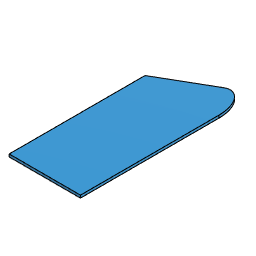
Nupud-T1 v1 (Autodesk Fusion 360 design; units mm, degrees)
Autodesk Fusion 360 part; units mm, degrees
sketch "Sketch1" plane through (0, 0, 0) normal (0, 0, 1) x (1, 0, 0)
  line L0 (-33, -71.5) -> (-33, -39.0517)
  spline S0 degree 3 poles (-33, -39.0517) (-33, -37.2602) (-33.4854, -35.4836) (-34.2537, -34.2725) (-34.9261, -33.2125) (-35.7722, -32.611) (-36.5563, -32.4575) (-37.1254, -32.346) (-37.6904, -32.44) (-38.2678, -32.7734) knots -1.570796 -1.570796 -1.570796 -1.570796 -0.801145 -0.801145 -0.801145 -0.12753 -0.12753 -0.12753 0.361367 0.361367 0.361367 0.361367
  line L1 (-38.2678, -32.7734) -> (-50, -39.547)
  line L2 (-50, -39.547) -> (-50, -71.5)
  line L3 (-50, -71.5) -> (-33, -71.5)
  line L4 (-33.2, -71.3) -> (-33.2, -39.0517)
  spline S1 degree 3 poles (-33.2, -39.0517) (-33.2, -37.2964) (-33.6813, -35.5482) (-34.4225, -34.3796) (-35.0726, -33.3548) (-35.8807, -32.7936) (-36.5947, -32.6537) (-37.1185, -32.5512) (-37.6252, -32.6333) (-38.1678, -32.9466) knots -1.570796 -1.570796 -1.570796 -1.570796 -0.801145 -0.801145 -0.801145 -0.12753 -0.12753 -0.12753 0.361367 0.361367 0.361367 0.361367
  line L5 (-38.1678, -32.9466) -> (-49.8, -39.6625)
  line L6 (-49.8, -39.6625) -> (-49.8, -71.3)
  line L7 (-49.8, -71.3) -> (-33.2, -71.3)
  dimension "d1" = 17
  dimension "d2" = 71.5
  dimension "d3" = 39.0517
  dimension "d4" = 33
  dimension "d5" = 120
  dimension "d6" = 6.2783
  dimension "d7" = -0.2
  constraint vertical L2
  constraint vertical L0
  constraint horizontal L3
  measures "d1" distance of L0 L2
  measures "d2" distance of origin L3
  measures "d3" vertical distance of origin L0.end
  measures "d4" distance of origin L0
  measures "d5" angle of L1 L2
  measures "d6" distance of L0.end S0.end
extrude "Extrude1" add sketch "Sketch1" along normal blind 0.6 contours L4 S1 L5 L6 L7
